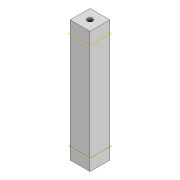
# Autodesk Inventor part: standoff for walls near wheel a
Saved by Autodesk Inventor 2020 (Build 240168000, 168)
## iProperties
Created: 2019-12-05
Part Number: standoff for walls near wheel a
Material: Generic
Document SubType Name: Modeling
Designer: ball
Density: 1 g/cm^3
Appearance: Default
Author: ball
Autodesk Inventor part; units mm, degrees
ref_plane "YZ Plane" through (0, 0, 0) normal (1, 0, 0) x (0, 1, 0)
ref_plane "XZ Plane" through (0, 0, 0) normal (0, 1, 0) x (-1, 0, 0)
ref_plane "XY Plane" through (0, 0, 0) normal (0, 0, 1) x (1, 0, 0)
sketch "Sketch1" plane through (0, 0, 0) normal (0, 1, 0) x (-1, 0, 0)
  line L0 (-6.35, 6.35) -> (6.35, 6.35)
  line L1 (6.35, 6.35) -> (6.35, -6.35)
  line L2 (6.35, -6.35) -> (-6.35, -6.35)
  line L3 (-6.35, -6.35) -> (-6.35, 6.35)
  line L4 (-6.35, 6.35) -> (6.35, -6.35) construction
  line L5 (6.35, 6.35) -> (-6.35, -6.35) construction
  circle A0 centre (0, 0) radius 1.7
  dimension "d0" = 12.7
  dimension "d1" = 12.7
  dimension "d2" = 3.4
  constraints: 12 end point, 2 midpoint, 2 parallel, 1 centre point, 1 coincident, 1 horizontal, 1 perpendicular
  measures "d0" distance of L1.end L2.end
  measures "d1" distance of L0.end L1.end
  measures "d2" diameter of A0
extrude "Extrusion1" add sketch "Sketch1" along normal blind 77.6732
ref_plane "Work Plane1" through (0, 69.9732, 0) normal (0, 1, 0) x (1, 0, 0)
sketch "Sketch2" plane through (0, 69.9732, 0) normal (0, 1, 0) x (1, 0, 0)
  circle A0 centre (0, 0) radius 1.7 construction
  circle A1 centre (0, 0) radius 3.45 construction
  line L0 (0, -3.45) -> (-2.9878, -1.725)
  line L1 (-2.9878, -1.725) -> (-2.9878, 6.35)
  line L2 (2.9878, 6.35) -> (2.9878, -1.725)
  line L3 (2.9878, -1.725) -> (0, -3.45)
  line L4 (6.35, 6.35) -> (-6.35, 6.35) projected
  line L5 (-2.9878, 6.35) -> (2.9878, 6.35)
  dimension "d6" = 6.9
  constraints: 10 end point, 2 coincident, 2 point on line, 1 vertical alignment, 8 other
extrude "Extrusion2" cut sketch "Sketch2" against normal blind 4.4
ref_plane "Work Plane2" through (0, 7.7, 0) normal (0, -1, 0) x (1, 0, 0)
sketch "Sketch3" plane through (0, 7.7, 0) normal (0, -1, 0) x (1, 0, 0)
  circle A0 centre (0, 0) radius 3.45 construction
  line L0 (2.9878, 1.725) -> (0, 3.45) projected
  line L1 (0, 3.45) -> (2.9878, 1.725)
  line L2 (2.9878, 1.725) -> (2.9878, -6.35)
  line L3 (-2.9878, -6.35) -> (-2.9878, 1.725)
  line L4 (-2.9878, 1.725) -> (0, 3.45)
  line L5 (6.35, -6.35) -> (-6.35, -6.35) projected
  line L6 (-2.9878, -6.35) -> (2.9878, -6.35)
  dimension "d10" = 6.9
  constraints: 10 end point, 2 coincident, 2 point on line, 1 centre point, 6 other
  measures "d10" diameter of A0
extrude "Extrusion3" cut sketch "Sketch3" against normal blind 4.4
body "Solid1"
